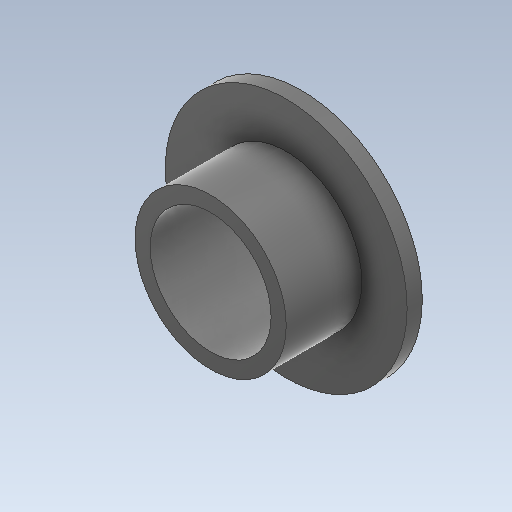
# Autodesk Inventor part: フランジブッシュ　d8-D10-l5-f16
Saved by Autodesk Inventor 2020 (Build 240168000, 168)
## iProperties
Created: 2020-02-26
Part Number: フランジブッシュ　d8-D10-l5-f16
Material: アセタール樹脂、黒
Document SubType Name: Modeling
Designer: tanjihayato
Density: 1.425 g/cm^3
Appearance: 滑らか - 黒
Mass: 0.41634 g
Surface Area: 6.59734 cm^2
Volume: 0.292168 cm^3
Author: tanjihayato
Autodesk Inventor part; units mm, degrees
ref_plane "YZ Plane" through (0, 0, 0) normal (1, 0, 0) x (0, 1, 0)
ref_plane "XZ Plane" through (0, 0, 0) normal (0, 1, 0) x (-1, 0, 0)
ref_plane "XY Plane" through (0, 0, 0) normal (0, 0, 1) x (1, 0, 0)
sketch "スケッチ1" plane through (0, 0, 0) normal (0, 0, 1) x (1, 0, 0)
  circle A0 centre (0, 0) radius 4
  circle A1 centre (0, 0) radius 5
  circle A2 centre (0, 0) radius 8
  dimension "d0" = 8
  dimension "d1" = 10
  dimension "d2" = 16
  constraints: 3 centre point, 3 coincident
  measures "d0" diameter of A0
  measures "d1" diameter of A1
  measures "d2" diameter of A2
extrude "押し出し1" add sketch "スケッチ1" along normal blind 1 contours A1 | A2
extrude "押し出し2" add sketch "スケッチ1" along normal blind 6 contours A1
